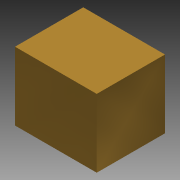
# Autodesk Inventor part: Gearmotor_Gear
Saved by Autodesk Inventor 2013 (Build 170138000, 138)
## iProperties
Created: 2015-07-02
Part Number: Gearmotor_Gear
Material: Brass, Soft Yellow
Document SubType Name: Modeling
Designer: Kyle
Density: 8.47 g/cm^3
Mass: 7.22501 g
Surface Area: 9.88055 cm^2
Volume: 0.853012 cm^3
Author: Kyle
Autodesk Inventor part; units mm, degrees
ref_plane "YZ Plane" through (0, 0, 0) normal (1, 0, 0) x (0, 1, 0)
ref_plane "XZ Plane" through (0, 0, 0) normal (0, 1, 0) x (-1, 0, 0)
ref_plane "XY Plane" through (0, 0, 0) normal (0, 0, 1) x (1, 0, 0)
sketch "Sketch1" plane through (0, 0, 0) normal (0, 0, 1) x (1, 0, 0)
  line L0 (0, 0) -> (11.9888, 0)
  line L1 (11.9888, 0) -> (11.9888, -10.0076)
  line L2 (11.9888, -10.0076) -> (0, -10.0076)
  line L3 (0, -10.0076) -> (0, 0)
  dimension "d0" = 10.0076
  dimension "d1" = 11.9888
  constraints: 8 end point, 2 parallel, 1 horizontal, 1 perpendicular
  measures "d0" distance of L2.end L0.start
  measures "d1" distance of L0.start L0.end
extrude "Extrusion1" add sketch "Sketch1" along normal blind 10.0076
shell "Shell1" thickness 1.27 removed faces 1 at (3.9963, -6.6717, 10.0076)
sketch "Sketch2" plane through (0, 0, 10.0076) normal (0, 0, 1) x (1, 0, 0)
  line L0 (1.27, -1.27) -> (10.7188, -1.27) projected
  line L1 (10.7188, -1.27) -> (10.7188, -8.7376) projected
  line L2 (10.7188, -8.7376) -> (1.27, -8.7376) projected
  line L3 (1.27, -8.7376) -> (1.27, -1.27) projected
extrude "Extrusion2" add sketch "Sketch2" against normal blind 3.81
body "Solid1"
